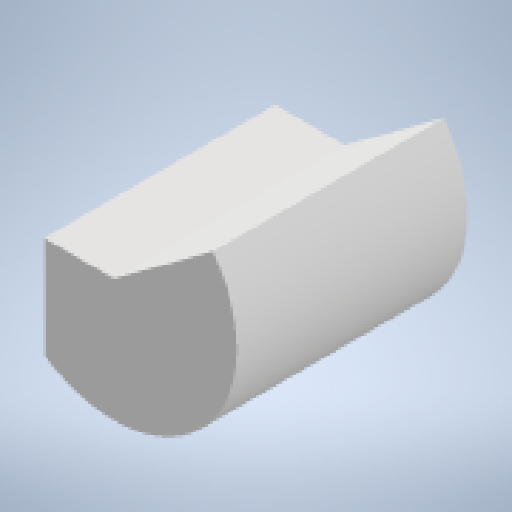
# Autodesk Inventor part: ROTATE
Saved by Autodesk Inventor 2023.2 (Build 272271030, 271C)
## iProperties
Created: 2023-06-22
Part Number: ROTATE
Material: Generic
Document SubType Name: Modeling
Designer: kao91
Density: 1 g/cm^3
Appearance: Default
Author: kao91
Autodesk Inventor part; units mm, degrees
ref_plane "YZ Plane" through (0, 0, 0) normal (1, 0, 0) x (0, 1, 0)
ref_plane "XZ Plane" through (0, 0, 0) normal (0, 1, 0) x (-1, 0, 0)
ref_plane "XY Plane" through (0, 0, 0) normal (0, 0, 1) x (1, 0, 0)
ref_plane "Work Plane1" through (-51.0014, -51.0767, 47.0039) normal (-0.0000478, 0, -1) x (0, 1, 0)
sketch "Sketch1" plane through (0, 0, 0) normal (0, 0, 1) x (1, 0, 0)
  arc A0 (-51.0012, -8.0945) -> (-16.6654, 27.298) centre (-36.8019, 12.4817) ccw
  line L0 (15.6535, 51.0767) -> (-36.8031, 12.4817) projected
  line L1 (-36.8031, 12.4817) -> (-51.0012, 12.4817) projected
  line L2 (-51.0012, 12.4817) -> (-51.0012, -51.0767) projected
  point P0 (0, 0)
  dimension "d0" = 50
  constraints: 2 point on circle, 2 point on line, 1 centre point
  measures "d0" diameter of A0
extrude "Extrusion1" add sketch "Sketch1" along normal up to surface (47.0015 mm away)
body "Solid1"
